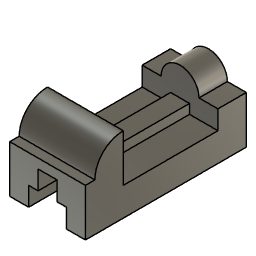
Task1b_2024A4PS0441P v1 (Autodesk Fusion 360 design; units mm, degrees)
Autodesk Fusion 360 part; units mm, degrees
sketch "Sketch1" plane through (0, 0, 0) normal (0, 0, 1) x (1, 0, 0)
  line L0 (0, 0) -> (40, 0)
  line L1 (0, 0) -> (0, 85)
  line L2 (0, 85) -> (40, 85)
  line L3 (40, 85) -> (40, 0)
  line L4 (0, 0) -> (0, 5)
  line L5 (0, 5) -> (40, 5)
  line L6 (40, 5) -> (40, 0)
  line L7 (0, 5) -> (0, 20)
  line L8 (0, 20) -> (40, 20)
  line L9 (40, 20) -> (40, 5)
  line L10 (0, 85) -> (0, 70)
  line L11 (0, 70) -> (40, 70)
  line L12 (40, 70) -> (40, 85)
  line L13 (0, 70) -> (15, 70)
  line L14 (15, 70) -> (15, 20)
  line L15 (15, 20) -> (25, 20)
  line L16 (15, 20) -> (25, 20)
  line L17 (25, 20) -> (25, 70)
  line L18 (25, 70) -> (15, 70)
  constraint coincident L0.start L1.start
  constraint horizontal L0
  constraint perpendicular L0 L1
  constraint perpendicular L1 L2
  constraint perpendicular L0 L3
  constraint coincident L1 L4.end
  constraint coincident L3 L5.end
  constraint perpendicular L3 L5
  constraint perpendicular L5 L7
  constraint coincident L3 L8.end
  constraint perpendicular L3 L8
  constraint perpendicular L2 L10
  constraint coincident L3 L11.end
  constraint perpendicular L3 L11
  constraint perpendicular L10 L13
  constraint coincident L8 L14.end
  constraint perpendicular L8 L14
  constraint coincident L8 L15.end
  constraint coincident L11 L17.end
  constraint perpendicular L11 L17
extrude "Extrude1" add sketch "Sketch1" along normal blind 25 contours L0 L1 L3 L4 L5 L6 makes body 1
extrude "Extrude2" add sketch "Sketch1" along normal blind 15 separate body contours L1 L8 L11 L13 L14 | L3 L8 L11 L17 makes body 2 at (0, 36.6667, 10) makes body 3 at (25, 36.6667, 10)
extrude "Extrude3" add sketch "Sketch1" along normal blind 20 contours L8 L11 L14 L15 L16 L17 L18 bodies 2 3
extrude "Extrude4" add sketch "Sketch1" along normal blind 25 contours L1 L2 L3 L10 L11 L12 L13 L18 bodies 2
extrude "Extrude5" add sketch "Sketch1" along normal blind 25 contours L1 L3 L5 L7 L8 L9 L15 L16 bodies 1 2
sketch "Sketch2" plane through (0, 0, 25) normal (0, 0, 1) x (-1, 0, 0)
  line L0 (0, 0) -> (-40, 0)
  line L1 (-40, 0) -> (-40, -20)
  line L2 (-40, -20) -> (0, -20)
  line L3 (0, -20) -> (0, 0)
  line L4 (0, -20) -> (0, -5)
  line L5 (-40, -5) -> (-40, -20)
  line L6 (0, -20) -> (-40, -20)
  line L7 (-40, -5) -> (0, -5)
  constraint coincident L2.end L3.start
  constraint coincident L3 L4.end
  constraint perpendicular L2 L4
  constraint coincident L1 L5.start
  constraint coincident L1.end L2.start
  constraint perpendicular L4 L7
sketch "Sketch3" plane through (40, 0, 0) normal (1, 0, 0) x (0, 1, 0)
  line L0 (0, 0) -> (85, 0)
  line L1 (85, 0) -> (85, 25)
  line L2 (85, 25) -> (70, 25)
  line L3 (70, 25) -> (70, 15)
  line L4 (70, 15) -> (20, 15)
  line L5 (20, 15) -> (20, 25)
  line L6 (20, 25) -> (0, 25)
  line L7 (0, 25) -> (0, 0)
  circle A0 centre (20, 25) radius 15
  line L8 (20, 25) -> (20, 40)
  constraint coincident L5.end L6.start
  constraint coincident A0 L8.end
  constraint perpendicular L6 L8
extrude "Extrude6" add sketch "Sketch3" against normal blind 40 contours L6 A0 L8 bodies 1
sketch "Sketch4" plane through (0, 85, 0) normal (0, 1, 0) x (-1, 0, 0)
  line L0 (-40, 0) -> (0, 0)
  line L1 (0, 0) -> (0, 25)
  line L2 (0, 25) -> (-40, 25)
  line L3 (-40, 25) -> (-40, 0)
  circle A0 centre (-20, 25) radius 10
  line L4 (-30, 25) -> (-10, 25)
  constraint midpoint L2 A0.centre
  constraint coincident L2 L4.start
  constraint coincident A0 L4.start
  constraint coincident A0 L4.end
  constraint coincident L2 L4.end
extrude "Extrude7" add sketch "Sketch4" against normal blind 15 contours L2 A0 L4 picked at (-23.1513, 27.4288) bodies 1
sketch "Sketch5" plane through (0, 0, 0) normal (0, -1, 0) x (1, 0, 0)
  line L0 (0, 0) -> (40, 0)
  line L1 (40, 0) -> (40, 25)
  line L2 (40, 25) -> (0, 25)
  line L3 (0, 25) -> (0, 0)
  line L4 (0, 0) -> (10, 0)
  line L5 (10, 0) -> (10, 10)
  line L6 (10, 10) -> (15, 10)
  line L7 (15, 10) -> (15, 20)
  line L8 (15, 20) -> (25, 20)
  line L9 (25, 20) -> (25, 10)
  line L10 (25, 10) -> (30, 10)
  line L11 (30, 10) -> (30, 0)
  line L12 (30, 0) -> (10, 0)
  constraint coincident L0.start L3.end
  constraint coincident L0 L4.end
  constraint perpendicular L3 L4
  constraint perpendicular L4 L5
  constraint perpendicular L5 L6
  constraint perpendicular L6 L7
  constraint perpendicular L7 L8
  constraint perpendicular L8 L9
  constraint perpendicular L9 L10
  constraint coincident L0 L11.end
  constraint perpendicular L0 L11
sketch "Sketch6" plane through (0, 0, 0) normal (0, -1, 0) x (1, 0, 0)
extrude "Extrude8" cut sketch "Sketch5" against normal blind 20 contours L0 L5 L6 L7 L8 L9 L10 L11 L12 bodies 1
